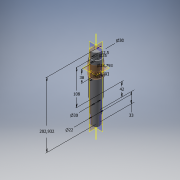
# Autodesk Inventor part: Вал быстроходный
Saved by Autodesk Inventor 2018 (Build 220112000, 112)
## iProperties
Created: 2018-03-24
Part Number: Вал быстроходный
Material: Типовые
Document SubType Name: Modeling
Designer: kriku
Density: 1 g/cm^3
Appearance: По умолчанию
Author: kriku
Autodesk Inventor part; units mm, degrees
sketch "Эскиз1" plane through (0, 0, 0) normal (1, 0, 0) x (0, 1, 0)
  point P0 (0, 0)
sketch "Эскиз2" plane through (0, 0, 0) normal (1, 0, 0) x (0, 1, 0)
  line L0 (0, 51.4323) -> (15, 51.4323)
  line L1 (15, 51.4323) -> (15, 31.5)
  line L2 (15, 31.5) -> (17.5, 31.5)
  line L3 (17.5, 31.5) -> (17.5, 19)
  line L4 (17.5, 19) -> (14.3965, 19)
  line L5 (14.3965, 19) -> (14.3965, -19)
  line L6 (14.3965, -19) -> (17.5, -19)
  line L7 (17.5, -19) -> (17.5, -76.5)
  line L8 (17.5, -76.5) -> (15, -76.5)
  line L9 (15, -76.5) -> (15, -118.5)
  line L10 (15, -118.5) -> (11, -118.5)
  line L11 (11, -118.5) -> (11, -151.5)
  line L12 (11, -151.5) -> (0, -151.5)
  line L13 (0, 51.4323) -> (0, -151.5)
  line L14 (16.2965, 19) -> (16.2965, -19)
  line L15 (18.8965, 19) -> (18.8965, -19)
  line L16 (18.8965, 19) -> (17.5, 19)
  line L17 (18.8965, -19) -> (17.5, -19)
  line L18 (0, 92.0188) -> (0, -192.0865) projected
  line L19 (-3.7793, 0) -> (22.6758, 0) projected
  point P0 (0, 0)
  dimension "d0" = 35
  dimension "d1" = 28.793
  dimension "d2" = 30
  dimension "d3" = 30
  dimension "d4" = 22
  dimension "d5" = 38
  dimension "d6" = 42
  dimension "d7" = 33
  dimension "d12" = 12.5
  dimension "d14" = 108
  dimension "d15" = 16.2965
  dimension "d17" = 37.793
  dimension "d21" = 202.9323
  constraints: 36 end point, 9 perpendicular, 4 vertical, 3 horizontal, 3 point on line, 2 horizontal alignment, 2 parallel, 1 collinear, 1 other
  measures "d0" diameter of L3 L13
  measures "d1" diameter of L5 L13
  measures "d2" diameter of L1 L13
  measures "d3" diameter of L9 L13
  measures "d4" diameter of L11 L13
  measures "d5" distance of L4.end L5.end
  measures "d6" distance of L8.end L9.end
  measures "d7" distance of L10.end L11.end
  measures "d12" distance of L2.end L3.end
  measures "d14" distance between parallel lines of L8 L2
  measures "d15" distance between parallel lines of L13 L14
  measures "d17" diameter of L15 L13
  measures "d21" distance between parallel lines of L12 L0
surface revolve "ВращПврх1" sketch "Эскиз2" angle 360 about axis through (0, 0, 51.4323) along (0, 0, -1) shown yes curves L16 L15 L17
revolve "Вращение1" add sketch "Эскиз2" angle 360 about axis through (0, 0, 51.4323) along (0, 0, -1) contours L0 L1 L2 L3 L4 L5 L19 L13 | L19 L5 L6 L7 L8 L9 L10 L11 L12 L13
surface revolve "ВращПврх2" sketch "Эскиз2" angle 360 about axis through (0, 0, 51.4323) along (0, 0, -1) shown yes curves L14
body "SRF1"
body "SRF2"
